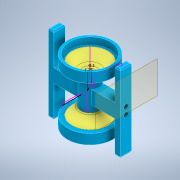
# Autodesk Inventor part: bistability_test_rack
Saved by Autodesk Inventor 2021 (Build 250183000, 183)
## iProperties
Created: 2021-01-14
Part Number: bistability_test_rack
Material: Generic
Document SubType Name: Modeling
Designer: Fierce PC
Density: 1 g/cm^3
Appearance: Default
Author: Fierce PC
Autodesk Inventor part; units mm, degrees
ref_plane "XZ Plane" through (0, 0, 0) normal (0, 1, 0) x (-1, 0, 0)
sketch "Sketch2" plane through (0, 0, 0) normal (0, 1, 0) x (-1, 0, 0)
  circle A0 centre (0, 0) radius 4
  circle A1 centre (0, 0) radius 2
  dimension "d0" = 8
  dimension "d1" = 4
  constraints: 2 centre point, 2 coincident
  measures "d0" diameter of A0
  measures "d1" diameter of A1
extrude "Extrusion1" add sketch "Sketch2" along normal blind 2 and the other way blind 3.5
sketch "Sketch3" plane through (0, 0, 0) normal (1, 0, 0) x (0, 1, 0)
  line L0 (2, -4) -> (2, 4) projected
  line L1 (-6.8114, 0) -> (9.3683, 0) projected
  line L2 (-3.5, 4) -> (2, 4) projected
  line L3 (-3.5, 4) -> (2, 4) projected
  arc A0 (2.2527, 4.61) -> (2, 4) centre (2.8627, 4) ccw
  line L4 (2, 4) -> (2, 2)
  line L5 (2, 2) -> (-3.5, 2) projected
  line L6 (3.0569, 2) -> (2, 2)
  line L7 (3.0569, 2) -> (3.0569, 4)
  line L8 (3.0569, 4) -> (7.0569, 8)
  line L9 (2.2527, 4.61) -> (5.6427, 8)
  line L10 (7.0569, 8) -> (5.6427, 8)
  point P0 (0, 0)
  dimension "d95" = 45
  dimension "d96" = 1
  dimension "d99" = 4
  constraints: 12 end point, 2 horizontal alignment, 2 point on circle, 2 point on line, 1 centre point, 1 horizontal, 1 parallel, 1 perpendicular, 1 tangent, 1 vertical
  measures "d96" distance between parallel lines of L8 L9
  measures "d99" horizontal distance of L7.end L8.end
revolve "Revolution1" add sketch "Sketch3" angle 360 about axis through (0, -10, 0) along (0, 1, 0) separate body
sketch "Sketch4" plane through (0, 0, 0) normal (0, 0, 1) x (1, 0, 0)
  line L0 (0, -6.8114) -> (0, 9.3683) projected
  line L1 (8, 7.0569) -> (-8, 7.0569) projected
  line L2 (8, 7.0569) -> (10, 7.0569)
  line L3 (10, 7.0569) -> (10, 5.6427)
  line L4 (10, 5.6427) -> (8, 5.6427)
  line L5 (8, 5.6427) -> (8, 7.0569)
  line L6 (4.61, 2.2527) -> (8, 5.6427) projected
  line L7 (8, 5.6427) -> (8, 7.0569) projected
  point P0 (0, 0)
  dimension "d98" = 10
  constraints: 8 end point, 2 parallel, 1 coincident, 1 horizontal, 1 perpendicular
  measures "d98" distance from line of L0 L2.end
revolve "Revolution2" add sketch "Sketch4" angle 360 about axis through (0, -10, 0) along (0, 1, 0) separate body
sketch "Sketch15" plane through (0, -3.5, 0) normal (0, -1, 0) x (1, 0, 0)
  circle A0 centre (0, 0) radius 2.7574 projected
  circle A1 centre (0, 0) radius 4
  dimension "d73" = 8
  constraints: 1 centre point, 1 coincident
  measures "d73" diameter of A1
extrude "Extrusion9" add sketch "Sketch15" along normal blind 0.5 contours A0 | A1 bodies 1
ref_plane "Work Plane6" through (0, 0, 0) normal (0.1736, 0, 0.9848) x (0, 1, 0)
ref_plane "Work Plane5" through (4.7625, 0, 0) normal (1, 0, 0) x (0, 1, 0)
sketch "Sketch21" plane through (0, 7.0569, 0) normal (0, 1, 0) x (1, 0, 0)
  arc A0 (-3.2392, 7.3149) -> (-5.022, 6.2273) centre (0, 0) ccw
  arc A1 (-3.6238, 8.1836) -> (-5.6184, 6.9668) centre (0, 0) ccw
  line L0 (-5.6184, 6.9668) -> (-5.022, 6.2273)
  line L1 (-3.2392, 7.3149) -> (-3.6238, 8.1836)
  dimension "d100" = 15
  dimension "d101" = 0.95
  constraints: 4 end point, 4 point on circle, 2 centre point, 1 coincident
  measures "d101" radial gap between concentric circles of A0 A1
extrude "Extrusion13" [suppressed]
sketch "Sketch23" plane through (-5.022, 7.0569, -6.2273) normal (-0.7784, 0, 0.6278) x (0.6278, 0, 0.7784)
  line L0 (-0.95, 2.3) -> (0, 2.3) projected
  line L1 (0, 0) -> (0, 2.3) projected
  line L2 (-0.95, 2.3) -> (0, 2.3)
  line L3 (0, 2.3) -> (0, 1.1)
  line L4 (0, 1.1) -> (-0.95, 1.1)
  line L5 (-0.95, 1.1) -> (-0.95, 2.3)
  line L6 (8, -14.3283) -> (8, 5.0714) projected
  point P0 (8, -7.0569)
  dimension "d105" = 1.2
  constraints: 8 end point, 2 parallel, 1 horizontal, 1 perpendicular, 1 point on line
  measures "d105" distance between parallel lines of L0 L4
revolve "Revolution3" [suppressed]
fillet "Fillet3" [suppressed]
pattern_circular "Circular Pattern5" [suppressed]
ref_plane "Work Plane8" through (16, 0, 0) normal (1, 0, 0) x (0, 1, 0)
sketch "Sketch26" plane through (16, 0, 0) normal (1, 0, 0) x (0, 1, 0)
  line L0 (-4, 4) -> (-4, -4) projected
  line L1 (-1, -2.475) -> (-4, -2.475)
  line L2 (-4, -2.475) -> (-4, 2.475)
  line L3 (-4, 2.475) -> (-1, 2.475)
  line L4 (-1, 2.475) -> (-1, -2.475)
  point P0 (0, 0)
  point P1 (-1, 0)
  point P2 (-4, -2.475)
  dimension "d115" = 4.95
  dimension "d117" = 3
  constraints: 8 end point, 2 parallel, 1 horizontal, 1 horizontal alignment, 1 midpoint, 1 perpendicular, 1 point on line
  measures "d115" distance of L3.end L1.start
  measures "d117" distance of L1.start L1.end
extrude "Extrusion14" add sketch "Sketch26" against normal up to next bodies 1
sketch "Sketch18" plane through (4.7625, 0, 0) normal (1, 0, 0) x (0, 1, 0)
  circle A0 centre (-2.4926, 0) radius 0.975
  line L0 (-4, 4) -> (-4, -4) projected
  point P0 (0, 0)
  dimension "d78" = 1.95
  dimension "d116" = 1.5074
  constraints: 1 centre point
  measures "d78" diameter of A0
  measures "d116" distance from line of L0 A0.centre
extrude "Extrusion10" cut sketch "Sketch18" along normal blind 12.1125 and the other way blind 3.675 bodies 1
pattern_circular "Circular Pattern6" count 2 over 360 about axis through (0, 6.3498, 0) along (0, -1, 0) of "Extrusion14" bodies 1
sketch "Sketch27" plane through (0, 7.0569, 0) normal (0, 1, 0) x (1, 0, 0)
  circle A0 centre (0, 0) radius 4.61 projected
  circle A1 centre (0, 0) radius 10
  circle A2 centre (0, 0) radius 9
  dimension "d125" = 1
  dimension "d128" = 20
  constraints: 2 centre point, 2 coincident
  measures "d125" radial gap between concentric circles of A1 A2
  measures "d128" diameter of A1
extrude "Extrusion15" add sketch "Sketch27" along normal blind 3 contours A1 bodies 3
sketch "Sketch28" plane through (-16, -1, 2.475) normal (0, 1, 0) x (1, 0, 0)
  line L0 (0, 4.95) -> (0, 0) projected
  line L1 (0, 4.95) -> (2.45, 4.95)
  line L2 (2.45, 4.95) -> (2.45, 0)
  line L3 (2.45, 0) -> (0, 0)
  line L4 (0, 0) -> (0, 4.95)
  line L5 (32, 4.95) -> (19.1424, 4.95) projected
  line L6 (32, 0) -> (19.1424, 0) projected
  line L7 (32, 4.95) -> (29.55, 4.95)
  line L8 (29.55, 4.95) -> (29.55, 0)
  line L9 (29.55, 0) -> (32, 0)
  line L10 (32, 0) -> (32, 4.95)
  point P0 (16, 2.475)
  point P1 (0, 0)
  point P2 (32, 0)
  point P3 (0, 0)
  dimension "d129" = 2.45
  dimension "d130" = 2.45
  dimension "d133" = 4.95
  constraints: 16 end point, 4 parallel, 2 horizontal, 2 perpendicular, 1 point on line
  measures "d129" distance of L0.start L1.end
  measures "d130" distance between parallel lines of L10 L8
  measures "d133" distance of L1.end L2.end
extrude "Extrusion16" add sketch "Sketch28" along normal blind 14 bodies 1
mirror "Mirror3" about plane through (16, -4, -2.475) normal (0, -1, 0) bodies 3 2 1
sketch "Sketch19" plane through (4.7625, 0, 0) normal (1, 0, 0) x (0, 1, 0)
  line L0 (-1, 3) -> (-7, 3)
  line L1 (-7, 3) -> (-7, 6.2171)
  line L2 (-7, 6.2171) -> (-1, 6.2171)
  line L3 (-1, 6.2171) -> (-1, 3)
  line L4 (-1, -3) -> (-7, -3)
  line L5 (-7, -3) -> (-7, -7.1834)
  line L6 (-7, -7.1834) -> (-1, -7.1834)
  line L7 (-1, -7.1834) -> (-1, -3)
  point P0 (0, 0)
  dimension "d81" = 6
  dimension "d82" = 7
  dimension "d83" = 3
  dimension "d84" = 6
  dimension "d85" = 3
  constraints: 16 end point, 4 parallel, 2 horizontal, 2 perpendicular
  measures "d81" distance of L1.end L2.end
  measures "d82" horizontal distance of L0.end point (0, 0)
  measures "d83" distance from line of point (0, 0) L0
  measures "d84" distance of L5.end L6.end
  measures "d85" distance from line of L4 point (0, 0)
extrude "Extrusion11" [suppressed]
sketch "Sketch10" plane through (0, 0, 0) normal (1, 0, 0) x (0, 1, 0)
  line L0 (-3, 12.5) -> (-3, -12.5) projected
  line L1 (0, -1.25) -> (-1.2, -1.25)
  line L2 (-1.5, -1.55) -> (-1.5, -12.5)
  line L3 (-3, -12.5) -> (-4.5, -12.5) projected
  arc A0 (-1.2, -1.25) -> (-1.5, -1.55) centre (-1.2, -1.55) ccw
  line L4 (-3, 12.5) -> (-4.5, 12.5) projected
  line L5 (-3.75, 12.5) -> (-3.75, 1.55)
  line L6 (-4.05, 1.25) -> (-3, 1.25)
  line L7 (-3, 2) -> (-3, -2) projected
  line L8 (-5.6, 0) -> (12.6, 0) projected
  arc A1 (-4.05, 1.25) -> (-3.75, 1.55) centre (-4.05, 1.55) ccw
  point P0 (0, 0)
  dimension "d49" = 1.5
  dimension "d50" = 1.25
  dimension "d51" = 0.3
  dimension "d52" = 1.25
  dimension "d53" = 0.3
  constraints: 8 end point, 4 point on circle, 4 tangent, 2 centre point, 2 point on line, 1 horizontal, 1 midpoint, 1 perpendicular, 1 vertical, 2 other
  measures "d49" distance from line of L1.start L2
  measures "d50" distance of point (0, 0) L1.start
  measures "d51" radius of A0
  measures "d52" distance between parallel lines of L8 L6
  measures "d53" radius of A1
fillet "Fillet2" radius 2 2 edges at (0, 3.0569, -4) (0, -11.0569, -4)
fillet "Fillet4" radius 0.5 16 edges at (-13.55, 13, 0) (-16, 13, 0) (-14.775, 13, 2.475) (-14.775, 13, -2.475) (14.775, 13, 2.475) (16, 13, 0) (13.55, 13, 0) (14.775, 13, -2.475) (-13.55, -21, 0) (-14.775, -21, 2.475) (-16, -21, 0) (-14.775, -21, -2.475) (14.775, -21, 2.475) (16, -21, 0) (13.55, -21, 0) (14.775, -21, -2.475)
sketch "Sketch29" plane through (-13.55, -7, -2.475) normal (0, -1, 0) x (1, 0, 0)
  line L0 (1.735, 4.0833) -> (10.4124, 4.0833) construction
  line L1 (10.4124, 4.0833) -> (10.4124, -0.6099) construction
  line L2 (10.4124, -0.6099) -> (1.735, -0.6099) construction
  line L3 (1.735, -0.6099) -> (1.735, 4.0833) construction
  line L4 (19.8663, 4.0158) -> (27.5308, 4.0158) construction
  line L5 (27.5308, 4.0158) -> (27.5308, -0.2722) construction
  line L6 (27.5308, -0.2722) -> (19.8663, -0.2722) construction
  line L7 (19.8663, -0.2722) -> (19.8663, 4.0158) construction
  line L8 (3.6838, 0.9736) -> (2.1969, 0.9736)
  line L9 (2.1969, 0.9736) -> (2.1969, 1.2848)
  line L10 (2.1969, 1.2848) -> (2.7502, 1.2848)
  line L11 (2.7502, 1.2848) -> (2.7502, 3.3275)
  line L12 (2.7502, 3.3275) -> (2.1969, 3.3275)
  line L13 (2.1969, 3.3275) -> (2.1969, 3.6066)
  spline S0 degree 2 poles (2.1969, 3.6066) (2.5106, 3.6066) (2.807, 3.7845) (2.8267, 4.0315) knots 0 0 0 1 2 2 2
  line L14 (2.8267, 4.0315) -> (3.1429, 4.0315)
  line L15 (3.1429, 4.0315) -> (3.1429, 1.2848)
  line L16 (3.1429, 1.2848) -> (3.6838, 1.2848)
  line L17 (3.6838, 1.2848) -> (3.6838, 0.9736)
  line L18 (4.8991, 0.9736) -> (4.41, 0.9736)
  line L19 (4.41, 0.9736) -> (4.41, 1.5565)
  line L20 (4.41, 1.5565) -> (4.8991, 1.5565)
  line L21 (4.8991, 1.5565) -> (4.8991, 0.9736)
  spline S1 degree 2 poles (7.4111, 2.4976) (7.4111, 1.6776) (6.9344, 0.9094) (6.4379, 0.9094) knots 0 0 0 1 2 2 2
  spline S2 degree 2 poles (6.4379, 0.9094) (5.934, 0.9094) (5.4623, 1.6924) (5.4623, 2.4951) knots 0 0 0 1 2 2 2
  spline S3 degree 2 poles (5.4623, 2.4951) (5.4623, 3.3201) (5.939, 4.0833) (6.4379, 4.0833) knots 0 0 0 1 2 2 2
  spline S4 degree 2 poles (6.4379, 4.0833) (6.9393, 4.0833) (7.4111, 3.2929) (7.4111, 2.4976) knots 0 0 0 1 2 2 2
  spline S5 degree 2 poles (6.8875, 1.5689) (6.9467, 1.7195) (6.9961, 2.1839) (6.9961, 2.4976) knots 0 0 0 1 2 2 2
  spline S6 degree 2 poles (6.9961, 2.4976) (6.9961, 2.8113) (6.9467, 3.2732) (6.885, 3.4288) knots 0 0 0 1 2 2 2
  spline S7 degree 2 poles (6.885, 3.4288) (6.8232, 3.5844) (6.6083, 3.745) (6.4379, 3.745) knots 0 0 0 1 2 2 2
  spline S8 degree 2 poles (6.4379, 3.745) (6.2675, 3.745) (6.0476, 3.5844) (5.9834, 3.4239) knots 0 0 0 1 2 2 2
  spline S9 degree 2 poles (5.9834, 3.4239) (5.9217, 3.2682) (5.8772, 2.794) (5.8772, 2.4951) knots 0 0 0 1 2 2 2
  spline S10 degree 2 poles (5.8772, 2.4951) (5.8772, 2.174) (5.9167, 1.7442) (5.981, 1.5763) knots 0 0 0 1 2 2 2
  spline S11 degree 2 poles (5.981, 1.5763) (6.0402, 1.4182) (6.2601, 1.2478) (6.4379, 1.2478) knots 0 0 0 1 2 2 2
  spline S12 degree 2 poles (6.4379, 1.2478) (6.6059, 1.2478) (6.8257, 1.4083) (6.8875, 1.5689) knots 0 0 0 1 2 2 2
  line L22 (22.0498, 2.0151) -> (21.6867, 2.0151)
  line L23 (21.6867, 2.0151) -> (21.6867, 0.9678)
  line L24 (21.6867, 0.9678) -> (21.294, 0.9678)
  line L25 (21.294, 0.9678) -> (21.294, 2.0151)
  line L26 (21.294, 2.0151) -> (19.9478, 2.0151)
  line L27 (19.9478, 2.0151) -> (19.9478, 2.4449)
  line L28 (19.9478, 2.4449) -> (21.3113, 4.0158)
  line L29 (21.3113, 4.0158) -> (21.6867, 4.0158)
  line L30 (21.6867, 4.0158) -> (21.6867, 2.3436)
  line L31 (21.6867, 2.3436) -> (22.0498, 2.3436)
  line L32 (22.0498, 2.3436) -> (22.0498, 2.0151)
  line L33 (21.294, 2.3436) -> (21.294, 3.5342)
  line L34 (21.294, 3.5342) -> (20.2689, 2.3436)
  line L35 (20.2689, 2.3436) -> (21.294, 2.3436)
  spline S13 degree 2 poles (24.2234, 1.9361) (24.2234, 1.7162) (24.0826, 1.3408) (23.9542, 1.2025) knots 0 0 0 1 2 2 2
  spline S14 degree 2 poles (23.9542, 1.2025) (23.8257, 1.0642) (23.4429, 0.9036) (23.2058, 0.9036) knots 0 0 0 1 2 2 2
  spline S15 degree 2 poles (23.2058, 0.9036) (22.9884, 0.9036) (22.5636, 0.9999) (22.408, 1.0765) knots 0 0 0 1 2 2 2
  line L36 (22.408, 1.0765) -> (22.408, 1.5088)
  line L37 (22.408, 1.5088) -> (22.4376, 1.5088)
  spline S16 degree 2 poles (22.4376, 1.5088) (22.4845, 1.4742) (22.6599, 1.3853) (22.7661, 1.3457) knots 0 0 0 1 2 2 2
  spline S17 degree 2 poles (22.7661, 1.3457) (22.8871, 1.3037) (23.0872, 1.2568) (23.2132, 1.2568) knots 0 0 0 1 2 2 2
  spline S18 degree 2 poles (23.2132, 1.2568) (23.3367, 1.2568) (23.5689, 1.3457) (23.6528, 1.4421) knots 0 0 0 1 2 2 2
  spline S19 degree 2 poles (23.6528, 1.4421) (23.7294, 1.5335) (23.8085, 1.7755) (23.8085, 1.9385) knots 0 0 0 1 2 2 2
  spline S20 degree 2 poles (23.8085, 1.9385) (23.8085, 2.1016) (23.7195, 2.309) (23.6356, 2.3782) knots 0 0 0 1 2 2 2
  spline S21 degree 2 poles (23.6356, 2.3782) (23.5491, 2.4548) (23.2922, 2.519) (23.1366, 2.519) knots 0 0 0 1 2 2 2
  spline S22 degree 2 poles (23.1366, 2.519) (22.9687, 2.519) (22.6352, 2.4671) (22.5339, 2.4449) knots 0 0 0 1 2 2 2
  line L38 (22.5339, 2.4449) -> (22.5339, 4.0158)
  line L39 (22.5339, 4.0158) -> (24.2061, 4.0158)
  line L40 (24.2061, 4.0158) -> (24.2061, 3.6577)
  line L41 (24.2061, 3.6577) -> (22.9267, 3.6577)
  line L42 (22.9267, 3.6577) -> (22.9267, 2.845)
  spline S23 degree 2 poles (22.9267, 2.845) (23.0008, 2.8549) (23.144, 2.8623) (23.2033, 2.8623) knots 0 0 0 1 2 2 2
  spline S24 degree 2 poles (23.2033, 2.8623) (23.438, 2.8623) (23.7615, 2.7858) (23.9097, 2.6721) knots 0 0 0 1 2 2 2
  spline S25 degree 2 poles (23.9097, 2.6721) (24.0604, 2.5585) (24.2234, 2.2127) (24.2234, 1.9361) knots 0 0 0 1 2 2 2
  point P0 (13.55, 2.475)
  constraints: 4 other
extrude "Extrusion17" add sketch "Sketch29" along normal blind 0.5 separate body
body "Solid1"
body "Solid2"
body "Solid3"
body "Solid10"
